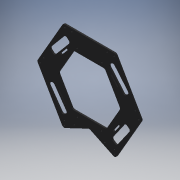
# Autodesk Inventor part: Bottom Plate
Saved by Autodesk Inventor 2017 (Build 210142000, 142)
## iProperties
Created: 2016-10-01
Part Number: Bottom Plate
Material: PVC, Unplasticized
Document SubType Name: Modeling
Designer: James Yelland
Density: 1.29 g/cm^3
Appearance: Smooth - White
Mass: 37.5584 g
Surface Area: 327.952 cm^2
Volume: 29.115 cm^3
Author: James Yelland
Autodesk Inventor part; units mm, degrees
ref_plane "YZ Plane" through (0, 0, 0) normal (1, 0, 0) x (0, 1, 0)
ref_plane "XZ Plane" through (0, 0, 0) normal (0, 1, 0) x (-1, 0, 0)
ref_plane "XY Plane" through (0, 0, 0) normal (0, 0, 1) x (1, 0, 0)
sketch "Sketch1" plane through (0, 0, 0) normal (0, 1, 0) x (-1, 0, 0)
  line L0 (103.5566, -2.5) -> (54.8095, -86.9325)
  line L1 (-54.8095, -86.9325) -> (-103.5566, -2.5)
  line L2 (-103.5566, 2.5) -> (-53.9434, 88.4327)
  line L3 (-49.6132, 90.9327) -> (49.6132, 90.9327)
  line L4 (53.9434, 88.4327) -> (103.5566, 2.5)
  line L5 (2.1497, -66.9563) -> (48.3297, -88.9468)
  line L6 (-2.1497, -66.9563) -> (-48.3297, -88.9468)
  arc A0 (48.3297, -88.9468) -> (54.8095, -86.9325) centre (50.4794, -84.4325) ccw
  arc A1 (2.1497, -66.9563) -> (-2.1497, -66.9563) centre (0, -71.4706) ccw
  arc A2 (-54.8095, -86.9325) -> (-48.3297, -88.9468) centre (-50.4794, -84.4325) ccw
  arc A3 (-103.5566, 2.5) -> (-103.5566, -2.5) centre (-99.2265, 0) ccw
  arc A4 (-49.6132, 90.9327) -> (-53.9434, 88.4327) centre (-49.6132, 85.9327) ccw
  arc A5 (53.9434, 88.4327) -> (49.6132, 90.9327) centre (49.6132, 85.9327) ccw
  arc A6 (103.5566, -2.5) -> (103.5566, 2.5) centre (99.2265, 0) ccw
  circle A7 centre (49.6132, 85.9327) radius 1.6
  circle A8 centre (-49.6132, 85.9327) radius 1.6
  circle A9 centre (-99.2265, 0) radius 1.6
  circle A10 centre (99.2265, 0) radius 1.6
  circle A11 centre (-25, 62.282) radius 1.6
  circle A12 centre (25, 62.282) radius 1.6
  circle A13 centre (24, -57.282) radius 1.6
  circle A14 centre (-24, -57.282) radius 1.6
  circle A15 centre (50.4794, -84.4325) radius 1.45
  circle A16 centre (50.4794, -76.4325) radius 1.45
  circle A17 centre (-50.4794, -76.4325) radius 1.45
  circle A18 centre (-50.4794, -84.4325) radius 1.45
  circle A19 centre (-30.6147, -73.9104) radius 1.6
  circle A20 centre (30.6147, -73.9104) radius 1.6
  circle A21 centre (35.5991, 85.9437) radius 1.6
  circle A22 centre (-35.5945, 85.9327) radius 1.6
  circle A23 centre (92.2171, 12.1406) radius 1.6
  circle A24 centre (-92.2171, 12.1406) radius 1.6
  arc A25 (31.3397, -49.282) -> (35.6699, -46.782) centre (31.3397, -44.282) ccw
  line L7 (31.3397, -49.282) -> (-31.3397, -49.282)
  arc A26 (-35.6699, -46.782) -> (-31.3397, -49.282) centre (-31.3397, -44.282) ccw
  line L8 (-35.6699, -46.782) -> (-61.2361, -2.5)
  arc A27 (-61.2361, 2.5) -> (-61.2361, -2.5) centre (-56.906, 0) ccw
  line L9 (-61.2361, 2.5) -> (-32.7831, 51.782)
  arc A28 (-28.453, 54.282) -> (-32.7831, 51.782) centre (-28.453, 49.282) ccw
  line L10 (-28.453, 54.282) -> (28.453, 54.282)
  arc A29 (32.7831, 51.782) -> (28.453, 54.282) centre (28.453, 49.282) ccw
  line L11 (32.7831, 51.782) -> (61.2361, 2.5)
  arc A30 (61.2361, -2.5) -> (61.2361, 2.5) centre (56.906, 0) ccw
  line L12 (61.2361, -2.5) -> (35.6699, -46.782)
  arc A31 (67.8361, 29.5077) -> (73.4714, 29.0147) centre (70.9003, 32.0789) ccw
  arc A32 (77.3017, 32.2286) -> (77.7947, 37.8639) centre (74.7305, 35.2928) ccw
  line L13 (73.4714, 29.0147) -> (77.3017, 32.2286)
  arc A33 (50.7976, 70.0378) -> (45.1623, 70.5308) centre (47.7335, 67.4666) ccw
  line L14 (45.1623, 70.5308) -> (41.3321, 67.3169)
  arc A34 (41.3321, 67.3169) -> (40.8391, 61.6815) centre (43.9032, 64.2527) ccw
  line L15 (64.2962, 53.9509) -> (50.7976, 70.0378)
  line L16 (64.2962, 53.9509) -> (77.7947, 37.8639)
  line L17 (40.8391, 61.6815) -> (67.8361, 29.5077)
  line L18 (49.7796, 41.77) -> (43.3517, 49.4305)
  line L19 (43.3517, 49.4305) -> (45.6499, 51.3589)
  line L20 (45.6499, 51.3589) -> (58.5056, 36.038)
  line L21 (58.5056, 36.038) -> (56.2075, 34.1096)
  line L22 (56.2075, 34.1096) -> (49.7796, 41.77)
  arc A35 (75.7207, -22.5008) -> (70.1497, -23.4831) centre (73.4264, -25.7774) ccw
  line L23 (58.1046, -40.6853) -> (60.9725, -36.5895)
  line L24 (49.9524, -47.1848) -> (61.4239, -30.8017)
  line L25 (61.4239, -30.8017) -> (58.9665, -29.081)
  line L26 (46.0596, -57.8875) -> (70.1497, -23.4831)
  line L27 (68.7536, -48.1418) -> (80.7987, -30.9396)
  line L28 (75.7207, -22.5008) -> (79.8164, -25.3687)
  arc A36 (80.7987, -30.9396) -> (79.8164, -25.3687) centre (77.5221, -28.6453) ccw
  line L29 (47.4949, -45.464) -> (49.9524, -47.1848)
  line L30 (53.2307, -37.2725) -> (47.4949, -45.464)
  arc A37 (51.1376, -66.3263) -> (56.7085, -65.344) centre (53.4319, -63.0497) ccw
  line L31 (68.7536, -48.1418) -> (56.7085, -65.344)
  line L32 (51.1376, -66.3263) -> (47.0419, -63.4584)
  arc A38 (46.0596, -57.8875) -> (47.0419, -63.4584) centre (49.3362, -60.1818) ccw
  line L33 (58.9665, -29.081) -> (53.2307, -37.2725)
  line L34 (-46.0596, -57.8875) -> (-70.1497, -23.4831)
  arc A39 (-70.1497, -23.4831) -> (-75.7207, -22.5008) centre (-73.4264, -25.7774) ccw
  line L35 (-61.4239, -30.8017) -> (-58.9665, -29.081)
  line L36 (-49.9524, -47.1848) -> (-61.4239, -30.8017)
  line L37 (-68.7536, -48.1418) -> (-80.7987, -30.9396)
  line L38 (-75.7207, -22.5008) -> (-79.8164, -25.3687)
  arc A40 (-79.8164, -25.3687) -> (-80.7987, -30.9396) centre (-77.5221, -28.6453) ccw
  line L39 (-47.4949, -45.464) -> (-49.9524, -47.1848)
  line L40 (-53.2307, -37.2725) -> (-47.4949, -45.464)
  line L41 (-58.9665, -29.081) -> (-53.2307, -37.2725)
  line L42 (-51.1376, -66.3263) -> (-47.0419, -63.4584)
  arc A41 (-56.7085, -65.344) -> (-51.1376, -66.3263) centre (-53.4319, -63.0497) ccw
  line L43 (-68.7536, -48.1418) -> (-56.7085, -65.344)
  arc A42 (-47.0419, -63.4584) -> (-46.0596, -57.8875) centre (-49.3362, -60.1818) ccw
  line L44 (-40.8391, 61.6815) -> (-67.8361, 29.5077)
  arc A43 (-73.4714, 29.0147) -> (-67.8361, 29.5077) centre (-70.9003, 32.0789) ccw
  line L45 (-73.4714, 29.0147) -> (-77.3017, 32.2286)
  arc A44 (-77.7947, 37.8639) -> (-77.3017, 32.2286) centre (-74.7305, 35.2928) ccw
  line L46 (-64.2962, 53.9509) -> (-77.7947, 37.8639)
  line L47 (-56.2075, 34.1096) -> (-49.7796, 41.77)
  line L48 (-49.7796, 41.77) -> (-43.3517, 49.4305)
  line L49 (-45.6499, 51.3589) -> (-58.5056, 36.038)
  line L50 (-58.5056, 36.038) -> (-56.2075, 34.1096)
  line L51 (-64.2962, 53.9509) -> (-50.7976, 70.0378)
  line L52 (-43.3517, 49.4305) -> (-45.6499, 51.3589)
  line L53 (-45.1623, 70.5308) -> (-41.3321, 67.3169)
  arc A45 (-45.1623, 70.5308) -> (-50.7976, 70.0378) centre (-47.7335, 67.4666) ccw
  arc A46 (-40.8391, 61.6815) -> (-41.3321, 67.3169) centre (-43.9032, 64.2527) ccw
  point P0 (105, 0)
  point P1 (52.5, -90.9327)
  point P2 (-105, 0)
  point P3 (-52.5, 90.9327)
  point P4 (52.5, 90.9327)
  point P5 (70.4073, 26.4435)
  point P6 (80.3658, 34.7998)
  point P7 (38.2679, 64.7457)
  point P8 (48.2265, 73.102)
  point P9 (54.3376, 45.5946)
  point P10 (57.5515, 41.7644)
  point P11 (72.4441, -20.2065)
  point P12 (54.4142, -68.6206)
  point P13 (43.7652, -61.1641)
  point P14 (83.093, -27.663)
  point P15 (-72.4441, -20.2065)
  point P16 (-83.093, -27.663)
  point P17 (-54.4142, -68.6206)
  point P18 (-70.4073, 26.4435)
  point P19 (-80.3658, 34.7998)
  point P20 (-48.2265, 73.102)
  point P21 (-38.2679, 64.7457)
  dimension "d11" = 360
  dimension "d30" = 360
  dimension "d90" = 360
  dimension "d136" = 360
  constraints: 108 end point, 58 point on circle, 53 centre point, 41 point on line, 6 coincident, 1 midpoint
extrude "Extrusion1" add sketch "Sketch1" along normal blind 3
body "Solid1"
